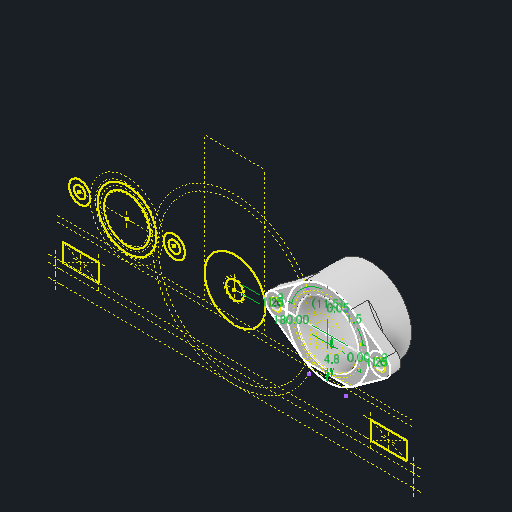
# Autodesk Inventor part: motorsupporter
Saved by Autodesk Inventor 2023.5 (Build 275446000, 446)
## iProperties
Created: 2025-01-19
Part Number: motorsupporter
Material: 一般
Document SubType Name: Modeling
Designer: IshiiLabHonda
Density: 1 g/cm^3
Appearance: 既定
Author: IshiiLabHonda
Autodesk Inventor part; units mm, degrees
ref_plane "YZ Plane" through (0, 0, 0) normal (1, 0, 0) x (0, 1, 0)
ref_plane "XZ Plane" through (0, 0, 0) normal (0, 1, 0) x (-1, 0, 0)
ref_plane "XY Plane" through (0, 0, 0) normal (0, 0, 1) x (1, 0, 0)
derived "motormount-l.ipt"
sketch "スケッチ2" plane through (0, 0, 0) normal (0, 0, 1) x (1, 0, 0)
  circle A0 centre (-15.0669, 1) radius 4.35 construction
  line L0 (0, 0) -> (0, 1) construction
  circle A1 centre (0, 0) radius 10.65 construction
  circle A2 centre (0, 0) radius 11.5 construction
  line L1 (-25, -8.7) -> (25, -8.7) construction
  line L2 (-25, -9.7) -> (25, -9.7) construction
  line L3 (-25, -11.5) -> (25, -11.5) construction
  line L4 (0, 0) -> (1, 0) construction
  circle A3 centre (12.9534, 1.1) radius 2.25 construction
  circle A4 centre (12.9534, 1.1) radius 4.25 construction
  circle A5 centre (-15.0669, 1) radius 3.6 construction
  circle A6 centre (-15.0669, 1) radius 3 construction
  circle A7 centre (0, 0) radius 1.25 construction
  circle A8 centre (0, 0) radius 1.5 construction
sketch "スケッチ3" plane through (0, 0, 0) normal (0, 0, 1) x (1, 0, 0)
  circle A0 centre (-15.0669, 1) radius 4.35 construction
  line L0 (0, 0) -> (0, 1) construction
  line L1 (0, 0) -> (1, 0) construction
  line L2 (-25, -11.5) -> (25, -11.5) construction
  line L3 (-25, -9.7) -> (25, -9.7) construction
  line L4 (-25, -8.7) -> (25, -8.7) construction
  circle A1 centre (12.9534, 1.1) radius 2.25 construction
  circle A2 centre (0, 0) radius 10.65 construction
  circle A3 centre (0, 0) radius 11.5 construction
  circle A4 centre (-15.0669, 1) radius 4.35 construction
  line L5 (0, 0) -> (0, 1) construction
  circle A5 centre (0, 0) radius 10.65 construction
  circle A6 centre (0, 0) radius 11.5 construction
  line L6 (-25, -8.7) -> (25, -8.7) construction
  line L7 (-25, -9.7) -> (25, -9.7) construction
  line L8 (-25, -11.5) -> (25, -11.5) construction
  line L9 (0, 0) -> (1, 0) construction
  circle A7 centre (12.9534, 1.1) radius 2.25 construction
  circle A8 centre (12.9534, 1.1) radius 4.25 construction
  circle A9 centre (-15.0669, 1) radius 3.6 construction
  circle A10 centre (-15.0669, 1) radius 3 construction
  line L10 (-24, -6.2) -> (-19, -6.2)
  line L11 (-19, -6.2) -> (-19, -8.7)
  line L12 (-24, -8.7) -> (-24, -6.2)
  line L13 (19, -6.2) -> (24, -6.2)
  line L14 (24, -6.2) -> (24, -8.7)
  line L15 (19, -8.7) -> (19, -6.2)
  line L16 (-24, -6.2) -> (-19, -8.7) construction
  line L17 (-24, -8.7) -> (-19, -6.2) construction
  line L18 (19, -6.2) -> (24, -8.7) construction
  line L19 (19, -8.7) -> (24, -6.2) construction
  line L20 (-24, -8.7) -> (-19, -8.7)
  line L21 (19, -8.7) -> (24, -8.7)
  circle A11 centre (-15.0669, 1) radius 3.2
  circle A12 centre (-15.0669, 1) radius 4.1
  circle A13 centre (12.9534, 1.1) radius 4.75 construction
  circle A14 centre (0, 0) radius 4.25
  circle A15 centre (0, 0) radius 1.25
  circle A16 centre (12.9534, 1.1) radius 1.5 construction
  line L22 (-4.25, 16.6) -> (-4.25, -3.4) construction
  line L23 (-4.25, 16.6) -> (4.25, 16.6) construction
  line L24 (4.25, 16.6) -> (4.25, -3.4) construction
  line L25 (-25, -3.4) -> (25, -3.4) construction
  line L26 (-25, -4.2) -> (25, -4.2) construction
  circle A17 centre (12.9534, 1.1) radius 5.75 construction
  circle A18 centre (20.2034, 1.1) radius 1.5
  circle A19 centre (20.2034, 1.1) radius 0.8
  circle A20 centre (5.7034, 1.1) radius 0.8
  circle A21 centre (5.7034, 1.1) radius 1.5
  line L27 (5.7034, 1.1) -> (12.9534, 1.1) construction
  line L28 (12.9534, 1.1) -> (20.2034, 1.1) construction
  circle A22 centre (-15.0669, 1) radius 5.1 construction
  circle A23 centre (-21.6669, 1) radius 0.8
  circle A24 centre (-21.6669, 1) radius 1.5
  circle A25 centre (-8.4669, 1) radius 0.8
  circle A26 centre (-8.4669, 1) radius 1.5
  line L29 (-21.6669, 1) -> (-15.0669, 1) construction
  line L30 (-15.0669, 1) -> (-8.4669, 1) construction
  point P0 (-21.5, -7.45)
  point P1 (21.5, -7.45)
sketch "スケッチ5" plane through (0, 0, 0) normal (0, 0, 1) x (1, 0, 0)
  circle A0 centre (-15.0669, 1) radius 4.35 construction
  line L0 (0, 0) -> (0, 1) construction
  circle A1 centre (0, 0) radius 10.65 construction
  circle A2 centre (0, 0) radius 11.5 construction
  line L1 (-25, -8.7) -> (25, -8.7) construction
  line L2 (-25, -9.7) -> (25, -9.7) construction
  line L3 (-25, -11.5) -> (25, -11.5) construction
  line L4 (0, 0) -> (1, 0) construction
  circle A3 centre (12.9534, 1.1) radius 2.25 construction
  circle A4 centre (12.9534, 1.1) radius 4.25 construction
  circle A5 centre (-15.0669, 1) radius 3.6 construction
  circle A6 centre (-15.0669, 1) radius 3 construction
  circle A7 centre (0, 0) radius 1.25 construction
  circle A8 centre (0, 0) radius 1.5 construction
  circle A9 centre (0, 0) radius 10.65 construction
  line L5 (0, 0) -> (0, 1) construction
  line L6 (0, 0) -> (1, 0) construction
  circle A10 centre (12.9534, 1.1) radius 2.25 construction
  circle A11 centre (-15.0669, 1) radius 4.35 construction
  circle A12 centre (0, 0) radius 11.5 construction
  line L7 (-25, -11.5) -> (25, -11.5) construction
  line L8 (-25, -9.7) -> (25, -9.7) construction
  line L9 (-25, -8.7) -> (25, -8.7) construction
  circle A13 centre (12.9534, 1.1) radius 2.25 construction
  circle A14 centre (12.9534, 1.1) radius 1.5 construction
  circle A15 centre (12.9534, 1.1) radius 2.25 construction
  circle A16 centre (12.9534, 1.1) radius 4.75 construction
  line L10 (19, -8.7) -> (19, -6.2) projected
  line L11 (24, -6.2) -> (24, -8.7) projected
  line L12 (19, -6.2) -> (24, -8.7) construction
  line L13 (19, -8.7) -> (24, -8.7) projected
  line L14 (19, -8.7) -> (24, -6.2) construction
  line L15 (19, -6.2) -> (24, -6.2) projected
  circle A17 centre (12.9534, 1.1) radius 4.25 construction
  circle A18 centre (-15.0669, 1) radius 4.35 construction
  line L16 (0, 0) -> (0, 1) construction
  line L17 (0, 0) -> (1, 0) construction
  line L18 (-25, -11.5) -> (25, -11.5) construction
  line L19 (-25, -9.7) -> (25, -9.7) construction
  line L20 (-25, -8.7) -> (25, -8.7) construction
  line L21 (0, 0) -> (0, 1) construction
  line L22 (0, 0) -> (1, 0) construction
  line L23 (-25, -8.7) -> (25, -8.7) construction
  line L24 (-25, -9.7) -> (25, -9.7) construction
  line L25 (-25, -11.5) -> (25, -11.5) construction
  circle A19 centre (0, 0) radius 11.5 construction
  circle A20 centre (0, 0) radius 11.5 construction
  circle A21 centre (0, 0) radius 10.65 construction
  circle A22 centre (0, 0) radius 10.65 construction
  circle A23 centre (0, 0) radius 1.25 projected
  circle A24 centre (0, 0) radius 4.25 projected
  circle A25 centre (-15.0669, 1) radius 4.35 construction
  circle A26 centre (-15.0669, 1) radius 3.6 construction
  circle A27 centre (-15.0669, 1) radius 3 construction
  circle A28 centre (-15.0669, 1) radius 3.2 projected
  circle A29 centre (-15.0669, 1) radius 4.1 projected
  line L26 (-19, -6.2) -> (-19, -8.7) projected
  line L27 (-24, -6.2) -> (-19, -6.2) projected
  line L28 (-24, -6.2) -> (-19, -8.7) construction
  line L29 (-24, -8.7) -> (-19, -6.2) construction
  line L30 (-24, -8.7) -> (-19, -8.7) projected
  line L31 (-24, -8.7) -> (-24, -6.2) projected
  circle A30 centre (12.9534, 1.1) radius 5.75
  circle A31 centre (20.2034, 1.1) radius 0.625
  circle A32 centre (20.2034, 1.1) radius 1.5
  circle A33 centre (20.2034, 1.1) radius 0.8 construction
  circle A34 centre (5.7034, 1.1) radius 0.625
  circle A35 centre (5.7034, 1.1) radius 1.5
  circle A36 centre (5.7034, 1.1) radius 0.8 construction
  circle A37 centre (12.9534, 1.1) radius 4.3
  line L32 (12.9534, 1.1) -> (20.2034, 1.1)
  line L33 (12.9534, 1.1) -> (5.7034, 1.1)
  line L34 (9.7875, -3.7) -> (16.1192, -3.7)
  line L35 (4.8241, 2.3152) -> (9.5827, 5.7584)
  line L36 (4.8241, -0.1152) -> (9.942, -3.8184)
  line L37 (12.9534, 1.1) -> (12.9534, 1.9)
  line L38 (21.0827, 2.3152) -> (16.3241, 5.7584)
  line L39 (21.0827, -0.1152) -> (16.3241, -3.5584)
  point P0 (21.5, -7.45)
  point P1 (-21.5, -7.45)
  point P2 (10.2336, 5.2463)
  point P3 (10.3436, -5.0259)
  point P4 (15.6732, 5.2463)
  point P5 (15.5631, -5.0259)
  point P6 (21.0827, 2.3152)
  point P7 (16.3698, 4.8084)
  point P8 (18.7034, 1.1)
  point P9 (16.3698, -4.5084)
  point P10 (21.0827, -0.1152)
  point P11 (9.5827, -3.5584)
  point P12 (7.2034, 1.1)
  point P13 (9.6284, 4.8084)
  dimension "d1" = 1.5
  dimension "d2" = 1.25
  dimension "d3" = 3
  dimension "d4" = 1.6
  dimension "d5" = 1.25
  dimension "d6" = 3
  dimension "d7" = 1.6
  dimension "d10" = 0.05
  dimension "d13" = 0
  dimension "d14" = 0
  dimension "d18" = 11.5
  dimension "d22" = 4.8
  constraints: 16 end point, 9 point on circle, 8 centre point, 8 tangent, 6 coincident, 4 symmetric about line, 1 parallel, 1 vertical, 13 other
  measures "d1" radial gap between concentric circles of A30 A4
  measures "d2" diameter of A31
  measures "d3" diameter of A32
  measures "d4" diameter of A33
  measures "d5" diameter of A34
  measures "d6" diameter of A35
  measures "d7" diameter of A36
  measures "d10" radial gap between concentric circles of A4 A37
  measures "d13" vertical extent of L32
  measures "d14" vertical extent of L33
  measures "d18" diameter of A30
  measures "d22" distance from line of A30.centre L34
extrude "押し出し1" add sketch "スケッチ5" against normal blind 1.5 contours A32 | A35
extrude "押し出し2" add sketch "スケッチ5" against normal blind 6 contours L32 A37 L33 A30 | A30 L34 L33 A37 L32 | A30 L34
extrude "押し出し3" cut sketch "スケッチ5" against normal blind 10 contours A30 L34
extrude "押し出し4" add sketch "スケッチ5" against normal blind 1.5 contours A32 L39 A30 | A30 L38 A32 | A30 A35 L35 | A30 L36 A35
fillet "フィレット1" radius 0.8 2 edges at (18.7034, 1.1, -1.5) (7.2034, 1.1, -1.5)
sketch "スケッチ1" plane through (0, 0, 0) normal (0, 0, 1) x (1, 0, 0)
  circle A0 centre (0, 0) radius 10.65 construction
  line L0 (0, 0) -> (0, 1) construction
  line L1 (0, 0) -> (1, 0) construction
  circle A1 centre (12.9534, 1.1) radius 2.25 construction
  circle A2 centre (-15.0669, 1) radius 4.35 construction
  circle A3 centre (0, 0) radius 11.5 construction
  line L2 (-25, -11.5) -> (25, -11.5) construction
  line L3 (-25, -9.7) -> (25, -9.7) construction
  line L4 (-25, -8.7) -> (25, -8.7) construction
  line L5 (-25, -4.2) -> (25, -4.2) construction
  line L6 (-25, -3.4) -> (25, -3.4) construction
  line L7 (-4.25, 16.6) -> (-4.25, -3.4) construction
  line L8 (4.25, 16.6) -> (4.25, -3.4) construction
  line L9 (-4.25, 16.6) -> (4.25, 16.6) construction
